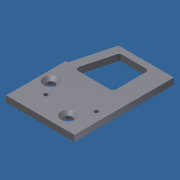
# Autodesk Inventor part: LATERAL-ESQUERDA
Saved by Autodesk Inventor 2012 SP1 (Build 160190100, 190)
## iProperties
Created: 2012-07-23
Part Number: LATERAL-ESQUERDA
Material: Carbon Steel
Document SubType Name: Modeling
Designer: bruno.silveira
Density: 7.87 g/cm^3
Mass: 130.183 g
Surface Area: 88.2317 cm^2
Volume: 16.5417 cm^3
Author: bruno.silveira
Autodesk Inventor part; units mm, degrees
ref_plane "YZ Plane" through (0, 0, 0) normal (1, 0, 0) x (0, 1, 0)
ref_plane "XZ Plane" through (0, 0, 0) normal (0, 1, 0) x (-1, 0, 0)
ref_plane "XY Plane" through (0, 0, 0) normal (0, 0, 1) x (1, 0, 0)
sketch "Sketch1" plane through (0, 0, 0) normal (0, 0, 1) x (1, 0, 0)
  line L0 (0, 0) -> (55, 0)
  line L1 (55, 0) -> (55, 80)
  line L2 (55, 80) -> (0, 80)
  line L3 (0, 80) -> (0, 0)
  dimension "d0" = 55
  dimension "d1" = 80
  constraints: 8 end point, 2 parallel, 1 horizontal, 1 perpendicular
  measures "d0" distance of L0.start L0.end
  measures "d1" distance of L2.end L0.start
extrude "Extrusion1" add sketch "Sketch1" along normal blind 5
sketch "Sketch6" plane through (0, 0, 5) normal (0, 0, 1) x (1, 0, 0)
  line L0 (0, 0) -> (0, 80) projected
  line L1 (55, 0) -> (0, 0) projected
  line L2 (0, 80) -> (55, 80) projected
  line L3 (0, 48) -> (2, 48)
  line L4 (2, 48) -> (10.5744, 80)
  dimension "d37" = 15
  dimension "d38" = 2
  dimension "d39" = 48
  constraints: 4 end point, 2 point on line, 1 parallel
  measures "d37" angle of L0 L4
  measures "d38" distance of L3.start L3.end
  measures "d39" distance between parallel lines of L1 L3
extrude "Extrusion4" cut sketch "Sketch6" against normal blind 5
sketch "Sketch7" plane through (0, 0, 5) normal (0, 0, 1) x (1, 0, 0)
  line L0 (10.5744, 80) -> (2, 48) projected
  line L1 (55, 80) -> (55, 0) projected
  line L2 (10.5744, 80) -> (55, 80) projected
  line L3 (40, 46) -> (40, 75)
  line L4 (40, 75) -> (16.4816, 75)
  line L5 (16.4816, 75) -> (8.711, 46)
  line L6 (8.711, 46) -> (40, 46)
  dimension "d42" = 29
  dimension "d43" = 5
  dimension "d44" = 15
  dimension "d45" = 7
  constraints: 8 end point, 2 parallel, 1 horizontal, 1 perpendicular
  measures "d42" distance of L3.start L3.end
  measures "d43" distance between parallel lines of L2 L4
  measures "d44" distance between parallel lines of L1 L3
  measures "d45" distance between parallel lines of L0 L5
extrude "Extrusion5" cut sketch "Sketch7" against normal blind 5
fillet "Fillet2" radius 2.5 4 edges at (16.4816, 75, 2.5) (40, 75, 2.5) (8.711, 46, 2.5) (40, 46, 2.5)
sketch "Sketch8" plane through (0, 0, 5) normal (0, 0, 1) x (1, 0, 0)
  line L0 (0, 0) -> (0, 48) projected
  line L1 (55, 0) -> (0, 0) projected
  line L2 (55, 80) -> (55, 0) projected
  point P0 (8, 28)
  point P1 (39, 11)
  dimension "d49" = 8
  dimension "d50" = 16
  dimension "d51" = 28
  dimension "d52" = 11
  measures "d49" distance from line of L0 point (8, 28)
  measures "d50" distance from line of L2 point (39, 11)
  measures "d51" distance from line of L1 point (8, 28)
  measures "d52" distance from line of L1 point (39, 11)
hole "Hole3" at (8, 28, 5) at (39, 11, 5) direction (0, 0, -1) diameter 6.5 depth 5 tip angle 118 countersink diameter 11.5 countersink angle 90
sketch "Sketch9" plane through (0, 0, 0) normal (0, 0, -1) x (-1, 0, 0)
  line L0 (-55, 0) -> (-55, 80) projected
  line L1 (0, 0) -> (-55, 0) projected
  line L2 (0, 48) -> (0, 0) projected
  point P0 (-15.5, 16.5)
  point P1 (-47.5, 25)
  dimension "d60" = 16.5
  dimension "d61" = 15.5
  dimension "d62" = 25
  dimension "d63" = 7.5
  measures "d60" distance from line of L1 point (-15.5, 16.5)
  measures "d61" distance from line of L2 point (-15.5, 16.5)
  measures "d62" distance from line of L1 point (-47.5, 25)
  measures "d63" distance from line of L0 point (-47.5, 25)
hole "Hole4" at (15.5, 16.5, 0) at (47.5, 25, 0) direction (0, 0, 1) diameter 3.175 depth 5 tip angle 118 countersink diameter 4 countersink angle 90
body "Solid1"
